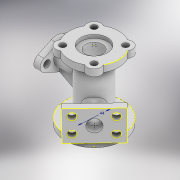
# Autodesk Inventor part: 2020216649-唐晨超-组合体2
Saved by Autodesk Inventor 2020 (Build 240168000, 168)
## iProperties
Created: 2021-03-17
Part Number: 2020216649-唐晨超-组合体2
Material: 常规
Document SubType Name: Modeling
Designer: Luorily
Density: 1 g/cm^3
Appearance: 默认
Author: Luorily
Autodesk Inventor part; units mm, degrees
ref_plane "YZ Plane" through (0, 0, 0) normal (1, 0, 0) x (0, 1, 0)
ref_plane "XZ Plane" through (0, 0, 0) normal (0, 1, 0) x (-1, 0, 0)
ref_plane "XY Plane" through (0, 0, 0) normal (0, 0, 1) x (1, 0, 0)
sketch "草图1" plane through (0, 0, 0) normal (1, 0, 0) x (0, 1, 0)
  point P0 (0, 0)
sketch "草图2" plane through (0, 0, 0) normal (0, 1, 0) x (-1, 0, 0)
  circle A0 centre (0, 0) radius 42
  dimension "d0" = 84
  constraints: 1 centre point, 1 coincident
  measures "d0" diameter of A0
extrude "拉伸1" add sketch "草图2" against normal blind 9
sketch "草图3" plane through (0, 0, 0) normal (0, 1, 0) x (1, 0, 0)
  circle A0 centre (0, 0) radius 42 projected
  circle A1 centre (0, 0) radius 22
  dimension "d3" = 44
  constraints: 1 centre point, 1 coincident
  measures "d3" diameter of A1
extrude "拉伸2" add sketch "草图3" along normal blind 81 contours A1
sketch "草图4" plane through (0, 81, 0) normal (0, 1, 0) x (1, 0, 0)
  circle A0 centre (0, 0) radius 22 projected
  line L0 (0, 0) -> (98.1595, 0) construction
  arc A1 (17.5955, -31.407) -> (31.407, -17.5955) centre (22.981, -22.981) ccw
  arc A2 (31.407, 17.5955) -> (17.5955, 31.407) centre (22.981, 22.981) ccw
  arc A3 (-17.5955, 31.407) -> (-31.407, 17.5955) centre (-22.981, 22.981) ccw
  arc A4 (-31.407, -17.5955) -> (-17.5955, -31.407) centre (-22.981, -22.981) ccw
  arc A5 (-17.5955, -31.407) -> (17.5955, -31.407) centre (0, 0) ccw
  arc A6 (-31.407, 17.5955) -> (-31.407, -17.5955) centre (0, 0) ccw
  arc A7 (31.407, -17.5955) -> (31.407, 17.5955) centre (0, 0) ccw
  arc A8 (17.5955, 31.407) -> (-17.5955, 31.407) centre (0, 0) ccw
  dimension "d32" = 20
  dimension "d35" = 360
  constraints: 16 point on circle, 8 centre point, 2 end point, 1 coincident, 1 horizontal, 17 other
  measures "d32" diameter of A1
extrude "拉伸3" add sketch "草图4" along normal blind 10 contours A0 | A5 A4 A6 A3 A8 A2 A7 A1
sketch "草图5" plane through (0, 91, 0) normal (0, 1, 0) x (0, 0, -1)
  arc A0 (-17.5955, -31.407) -> (17.5955, -31.407) centre (0, 0) ccw projected
  constraints: 1 coincident
hole "孔2" at (0, 91, 0) direction (0, -1, 0) diameter 39 depth 5
sketch "草图6" plane through (0, 91, 0) normal (0, 1, 0) x (0, 0, -1)
  circle A0 centre (0, 0) radius 19.5 projected
  arc A1 (-17.5955, -31.407) -> (17.5955, -31.407) centre (0, 0) ccw projected
  line L0 (0, 0) -> (79.4975, 0) construction
  circle A2 centre (0, 0) radius 12.5 projected
  circle A3 centre (0, 0) radius 32.5
  circle A4 centre (22.981, 22.981) radius 4.5
  circle A5 centre (-22.981, 22.981) radius 4.5
  circle A6 centre (-22.981, -22.981) radius 4.5
  circle A7 centre (22.981, -22.981) radius 4.5
  dimension "d25" = 9
  dimension "d28" = 360
  constraints: 4 centre point, 3 coincident, 2 end point, 1 horizontal, 14 other
  measures "d25" diameter of A4
extrude "拉伸4" cut sketch "草图6" against normal blind 10 contours A4 A3 | A3 A4 | A7 A3 | A3 A7 | A5 A3 | A3 A5 | A6 A3 | A3 A6
sketch "草图10" plane through (0, 0, 0) normal (1, 0, 0) x (0, 1, 0)
  line L0 (-9, 42) -> (-9, -42) projected
  line L1 (-9, 0) -> (57, 0)
  circle A0 centre (57, 0) radius 14
  point P0 (0, 0)
  dimension "d43" = 66
  dimension "d44" = 28
  constraints: 2 end point, 1 centre point, 1 coincident, 1 horizontal, 1 midpoint
  measures "d43" distance of L1.start L1.end
  measures "d44" diameter of A0
extrude "拉伸5" add sketch "草图10" against normal blind 54
hole "孔3" at (0, 91, 0) direction (0, -1, 0) diameter 25 end through all
sketch "草图11" plane through (-54, 57, 0) normal (-1, 0, 0) x (0, 0, 1)
  circle A0 centre (0, 0) radius 14 projected
  circle A1 centre (24, 0) radius 5
  circle A2 centre (-24, 0) radius 5
  arc A3 (-28.1667, 9.0906) -> (-28.1667, -9.0906) centre (-24, 0) ccw
  arc A4 (28.1667, -9.0906) -> (28.1667, 9.0906) centre (24, 0) ccw
  line L0 (-28.1667, 9.0906) -> (-8.3333, 18.1812)
  line L1 (28.1667, 9.0906) -> (8.3333, 18.1812)
  line L2 (28.1667, -9.0906) -> (8.3333, -18.1812)
  line L3 (-28.1667, -9.0906) -> (-8.3333, -18.1812)
  arc A5 (-8.3333, -18.1812) -> (8.3333, -18.1812) centre (0, 0) ccw
  arc A6 (8.3333, 18.1812) -> (-8.3333, 18.1812) centre (0, 0) ccw
  point P0 (0, -57)
  dimension "d56" = 10
  dimension "d57" = 10
  dimension "d58" = 20
  dimension "d59" = 20
  constraints: 8 end point, 8 point on circle, 8 tangent, 6 centre point, 3 coincident
  measures "d56" diameter of A1
  measures "d57" diameter of A2
  measures "d58" diameter of A3
  measures "d59" diameter of A4
extrude "拉伸6" add sketch "草图11" against normal blind 9
sketch "草图12" plane through (-54, 0, 0) normal (-1, 0, 0) x (0, 0, 1)
  arc A0 (8.3333, 75.1812) -> (-8.3333, 75.1812) centre (0, 57) ccw projected
  point P0 (0, 0)
  constraints: 1 coincident
hole "孔4" at (-54, 57, 0) direction (1, 0, 0) diameter 18 end up to surface
ref_plane "工作平面8" through (31.407, 81, 17.5955) normal (0.7071068, 0, 0.7071068) x (0, 1, 0)
sketch "草图13" plane through (31.407, 81, 17.5955) normal (0.7071068, 0, 0.7071068) x (0, 1, 0)
  line L0 (-90, 51.7661) -> (-90, -32.2339) projected
  circle A0 centre (-54, 9.7661) radius 14
  point P0 (-81, 9.7661)
  dimension "d72" = 28
  constraints: 1 centre point
  measures "d72" diameter of A0
extrude "拉伸7" add sketch "草图13" against normal blind 18
sketch "草图14" plane through (24.5012, 27, 24.5012) normal (0.7071068, 0, 0.7071068) x (0.7071068, 0, -0.7071068)
  circle A0 centre (0, 0) radius 14 projected
  point P0 (0, -27)
extrude "拉伸8" add sketch "草图14" along normal blind 18
sketch "草图15" plane through (37.2292, 27, 37.2292) normal (0.7071068, 0, 0.7071068) x (0.7071068, 0, -0.7071068)
  circle A0 centre (0, 0) radius 14 projected
  line L0 (34, 0) -> (34, 22)
  line L1 (34, 22) -> (-33.9926, 21)
  line L2 (-8.8388, 21) -> (-38.1838, 21) projected
  line L3 (-33.9926, 21) -> (-33.3456, -22.9952)
  line L4 (-33.3456, -22.9952) -> (34, -22.0048)
  line L5 (34, -22.0048) -> (34, 0)
  line L6 (22, -27) -> (22, 54) projected
  line L7 (0, 0) -> (23, 0) construction
  circle A1 centre (23, 11) radius 5
  circle A2 centre (23, -11) radius 5
  circle A3 centre (-23, 11) radius 5
  circle A4 centre (-23, -11) radius 5
  point P0 (0, -27)
  dimension "d77" = 34
  dimension "d78" = 22
  dimension "d79" = 68
  dimension "d80" = 44
  dimension "d88" = 10
  constraints: 12 end point, 4 centre point, 2 perpendicular, 2 point on line, 1 horizontal
  measures "d77" distance of L7.start L0.start
  measures "d78" distance of L0.start L0.end
  measures "d79" distance of L0.end L1.end
  measures "d80" distance of L1.end L3.end
  measures "d88" diameter of A1
extrude "拉伸9" add sketch "草图15" against normal blind 9 contours L5 L4 L6 A2 A1 L1 L0 | L6 A1 A2 L4 L3 L1
sketch "草图16" plane through (37.2292, 27, 37.2292) normal (0.7071068, 0, 0.7071068) x (0.7071068, 0, -0.7071068)
  circle A0 centre (-23, 11) radius 5 projected
  circle A1 centre (-23, -11) radius 5 projected
  circle A2 centre (23, 11) radius 5 projected
  circle A3 centre (23, -11) radius 5 projected
  line L0 (34, -22.0048) -> (34, 22) projected
  line L1 (34, 22) -> (-33.9926, 21) projected
  line L2 (-33.9926, 21) -> (-33.3456, -22.9952) projected
  line L3 (-33.3456, -22.9952) -> (34, -22.0048) projected
  point P0 (0, -27)
  point P1 (0.3272, -0.4976)
sketch "草图17" plane through (37.2292, 27, 37.2292) normal (0.7071068, 0, 0.7071068) x (0.7071068, 0, -0.7071068)
  point P0 (0, -27)
  point P1 (0.3272, -0.4976)
  point P2 (0.3272, -0.4976)
  constraints: 1 coincident
hole "孔5" at (37.4605, 26.5024, 36.9978) direction (-0.7071068, 0, -0.7071068) diameter 18 end up to surface
sketch "草图18" plane through (0, 0, 0) normal (0, 0, 1) x (1, 0, 0)
  line L0 (-54, 52) -> (-54, 62) projected
  line L1 (-45, 37) -> (-45, 38.8188) projected
  line L2 (-22, 25) -> (-45, 37)
  line L3 (-45, 37) -> (-45, 44.4162)
  line L4 (-45, 47.9094) -> (-45, 38.8188) projected
  line L5 (-22, 25) -> (-19.6996, 23.7998)
  line L6 (-19.6996, 23.7998) -> (-19.6996, 43.0992)
  line L7 (-22, 0) -> (-22, 81) projected
  point P0 (0, 0)
  constraints: 8 end point, 1 parallel, 1 point on line
extrude "加强筋1" add sketch "草图18" along normal mid plane 10 rib yes fills toward (-19.7496, 33.4495) open curves L6 L5 L2 L3
